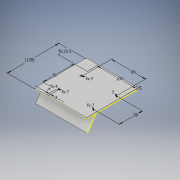
# Autodesk Inventor part: angle test
Saved by Autodesk Inventor 2019 (Build 230136000, 136)
## iProperties
Created: 2020-02-13
Part Number: angle test
Material: Generic
Document SubType Name: Modeling
Designer: close
Density: 1 g/cm^3
Appearance: Default
Author: close
Autodesk Inventor part; units mm, degrees
ref_plane "YZ Plane" through (0, 0, 0) normal (1, 0, 0) x (0, 1, 0)
ref_plane "XZ Plane" through (0, 0, 0) normal (0, 1, 0) x (-1, 0, 0)
ref_plane "XY Plane" through (0, 0, 0) normal (0, 0, 1) x (1, 0, 0)
sketch "Sketch1" plane through (0, 0, 0) normal (0, 1, 0) x (-1, 0, 0)
  line L0 (0, 0) -> (130, 0)
  line L1 (130, 0) -> (130, -130)
  line L2 (130, -130) -> (0, -130)
  line L3 (0, -130) -> (0, 0)
  dimension "d0" = 130
  dimension "d1" = 130
  constraints: 8 end point, 2 parallel, 1 horizontal, 1 perpendicular
  measures "d0" distance of L0.end L1.end
  measures "d1" distance of L1.end L2.end
extrude "Extrusion1" add sketch "Sketch1" along normal blind 2.5
sketch "Sketch2" plane through (0, 0, 0) normal (0, -1, 0) x (1, 0, 0)
  line L0 (-2.5, -104.5) -> (-102.5, -104.5) construction
  line L1 (-102.5, -104.5) -> (-102.5, -25.5) construction
  line L2 (-102.5, -25.5) -> (-2.5, -25.5) construction
  line L3 (-2.5, -25.5) -> (-2.5, -104.5) construction
  line L4 (-12.5, -87.5) -> (-98.5, -87.5) construction
  line L5 (-98.5, -87.5) -> (-98.5, -29.5) construction
  line L6 (-98.5, -29.5) -> (-12.5, -29.5) construction
  line L7 (-12.5, -29.5) -> (-12.5, -87.5) construction
  line L8 (0, 0) -> (-130, 0) construction
  line L9 (-130, -130) -> (0, -130) construction
  line L10 (-130, 0) -> (-130, -130) construction
  circle A0 centre (-12.5, -87.5) radius 3.5
  circle A1 centre (-98.5, -87.5) radius 3.5
  circle A2 centre (-12.5, -29.5) radius 3.5
  circle A3 centre (-98.5, -29.5) radius 3.5
  line L11 (0, -130) -> (0, 0) projected
  dimension "d4" = 86
  dimension "d5" = 58
  dimension "d6" = 100
  dimension "d7" = 79
  dimension "d8" = 4
  dimension "d9" = 4
  dimension "d10" = 130
  dimension "d11" = 25.5
  dimension "d13" = 7
  dimension "d14" = 7
  dimension "d15" = 7
  dimension "d16" = 7
  dimension "d27" = 2.5
  constraints: 16 end point, 8 coincident, 4 centre point, 4 parallel, 2 horizontal, 2 perpendicular
  measures "d4" distance of L4.start L4.end
  measures "d5" distance of L6.end L4.start
  measures "d6" distance of L0.start L0.end
  measures "d7" distance of L0.end L1.end
  measures "d8" distance from line of L1 L5.end
  measures "d9" distance between parallel lines of L2 L6
  measures "d10" distance between parallel lines of L8 L9
  measures "d11" distance between parallel lines of L0 L9
  measures "d13" diameter of A0
  measures "d14" diameter of A1
  measures "d15" diameter of A2
  measures "d16" diameter of A3
  measures "d27" distance between parallel lines of L11 L3
extrude "Extrusion2" add sketch "Sketch2" along normal blind 2.25
fillet "Fillet1" radius 1 4 edges at (-16, 0, -87.5) (-16, 0, -29.5) (-102, 0, -29.5) (-102, 0, -87.5)
sketch "Sketch3" plane through (-12.5, -2.25, -87.5) normal (0, -1, 0) x (1, 0, 0)
  circle A0 centre (0, 0) radius 3.5 construction
  circle A1 centre (-86, 0) radius 3.5 construction
  circle A2 centre (0, 58) radius 3.5 construction
  circle A3 centre (-86, 58) radius 3.5 construction
  circle A4 centre (0, 0) radius 4.5 construction
  circle A5 centre (-86, 58) radius 3.5 construction
  point P0 (12.5, 87.5)
  point P1 (0, 58)
  point P2 (-86, 58)
  constraints: 4 coincident
hole "Hole1" at (-12.5, -2.25, -87.5) at (-12.5, -2.25, -29.5) at (-98.5, -2.25, -29.5) at (-98.5, -2.25, -87.5) direction (0, 1, 0) diameter 2.013 depth 4.75 thread size "M2.5x0.45" class "6H" standard "ANSI Metric M Profile"
sketch "Sketch4" plane through (0, 0, 0) normal (1, 0, 0) x (0, 0, -1)
  line L0 (130, 0) -> (0, 0) projected
  line L1 (25.5, 0) -> (-8.1173, -48.0104) construction
  line L2 (25.5, 0) -> (2.5569, -32.7661)
  line L3 (2.5569, -32.7661) -> (1.7378, -32.1925)
  line L4 (1.7378, -32.1925) -> (24.2792, 0)
  line L5 (25.5, 0) -> (24.2792, 0)
  point P0 (25.5, 0)
  dimension "d28" = 55
  dimension "d29" = 0
  dimension "d30" = 1
  dimension "d31" = 40
  constraints: 10 end point, 3 point on line, 2 perpendicular, 1 horizontal
  measures "d28" angle of L1 L0
  measures "d29" distance of L1.start point (25.5, 0)
  measures "d30" distance between parallel lines of L1 L4
  measures "d31" distance of point (25.5, 0) L2.end
extrude "Extrusion3" add sketch "Sketch4" against normal blind 130
sketch "Sketch5" plane through (0, 2.5, 0) normal (1, 0, 0) x (0, 0, -1)
  line L0 (24.2792, -2.5) -> (1.7378, -34.6925) projected
  point P0 (0, -2.5)
equation "\"d9\" = d8"
equation "\"d11\" = -0.5 * d7 + 0.5 * d10"
equation "\"d14\" = d13"
equation "\"d15\" = d14"
equation "\"d16\" = d15"
body "Solid1"
